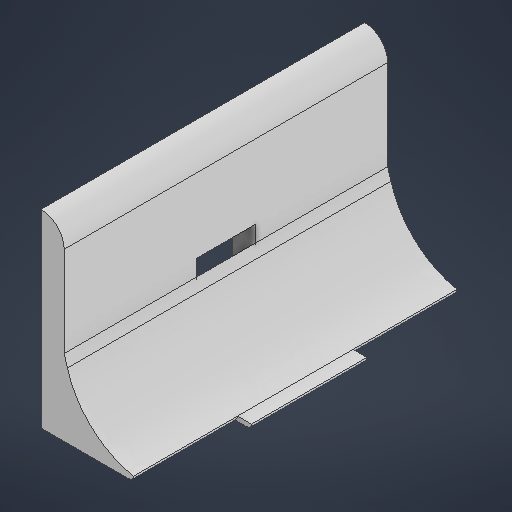
# Autodesk Inventor part: Ramp
Saved by Autodesk Inventor 2026.1 (Build 301233000, 233)
## iProperties
Created: 2026-05-11
Part Number: Ramp
Material: Generic
Document SubType Name: Modeling
Designer: 25adoh
Density: 1 g/cm^3
Appearance: Default
Author: 25adoh
Autodesk Inventor part; units mm, degrees
ref_plane "YZ Plane" through (0, 0, 0) normal (1, 0, 0) x (0, 1, 0)
ref_plane "XZ Plane" through (0, 0, 0) normal (0, 1, 0) x (-1, 0, 0)
ref_plane "XY Plane" through (0, 0, 0) normal (0, 0, 1) x (1, 0, 0)
sketch "Sketch1" plane through (0, 0, 0) normal (1, 0, 0) x (0, 1, 0)
  line L0 (-5, -70) -> (-5, 70)
  line L1 (-5, 70) -> (5, 70)
  line L2 (5, 70) -> (5, -70)
  line L3 (5, -70) -> (-5, -70)
  line L4 (-5, -70) -> (5, 70) construction
  line L5 (-5, 70) -> (5, -70) construction
  line L6 (5, 70) -> (75, 70)
  line L7 (75, 70) -> (75, -70)
  line L8 (75, -70) -> (5, -70)
  line L9 (5, -70) -> (5, 70)
  line L10 (5, -25) -> (5, 0.7)
  line L11 (75, 0.7) -> (75, -25)
  line L12 (35, 12.85) -> (-5, 12.85)
  line L13 (-5, 12.85) -> (-5, -12.85)
  line L14 (-5, -12.85) -> (35, -12.85)
  line L15 (35, -12.85) -> (35, 12.85)
  line L16 (35, 12.85) -> (-5, -12.85) construction
  line L17 (-5, 12.85) -> (35, -12.85) construction
  line L18 (35, -12.85) -> (-10, -12.85)
  line L19 (-10, -12.85) -> (-10, 12.85)
  line L20 (-10, 12.85) -> (35, 12.85)
  line L21 (35, 12.85) -> (35, -12.85)
  point P0 (0, 0)
  point P1 (40, -12.15)
  point P2 (15, 0)
  dimension "d0" = 140
  dimension "d1" = 10
  dimension "d2" = 70
  dimension "d29" = 25.7
  dimension "d30" = 45
  constraints: 44 end point, 9 parallel, 4 midpoint, 4 perpendicular, 3 horizontal, 2 point on line, 1 vertical
  measures "d0" distance of L0.start L0.end
  measures "d1" distance of L0.end L1.end
  measures "d2" distance of L7.end L8.end
  measures "d29" distance of L13.end L12.end
  measures "d30" distance of L19.end L20.end
extrude "Extrusion1" add sketch "Sketch1" along normal blind 10 contours L0 L14 L2 L3 | L0 L12 L2 L14 | L0 L1 L2 L12
extrude "Extrusion2" add sketch "Sketch1" along normal blind 4 contours L2 L14 L15 L12 L6 L7 L8 | L2 L12 L15 L14
extrude "Extrusion3" add sketch "Sketch1" along normal blind 10 contours L2 L14 L15 L12 L6 L7 L8 | L2 L12 L15 L14
sketch "Sketch2" plane through (0, -5, 70) normal (0, 0, 1) x (1, 0, 0)
  line L0 (4, 10) -> (4, 80) projected
  line L1 (10, 0) -> (10, 80) projected
  line L2 (10, 0) -> (20, 0)
  line L3 (10, 10) -> (10, 80) projected
  line L4 (4, 80) -> (4, 0)
  line L5 (4, 0) -> (20, 0)
  line L6 (0, 0) -> (40, 0)
  arc A0 (4, 80) -> (11.3887, 26.2221) centre (170.9276, 75.538) ccw
  arc A1 (11.3887, 26.2221) -> (40, 0) centre (47.0584, 36.4217) ccw
  line L7 (4, 71.0761) -> (4, 0)
  line L8 (4, 0) -> (40, 0)
  line L9 (40, 0) -> (45, 0)
  line L10 (15, 0) -> (25, 0)
  line L11 (9, 0) -> (25, 0)
  line L12 (5, 0) -> (45, 0)
  line L13 (9, 0) -> (45, 0)
  point P0 (0, 5)
  point P1 (10, 38.164)
  point P2 (4, 71.0761)
  point P3 (66.442, 18.3754)
  point P4 (9, 10)
  point P5 (15, 38.164)
  point P6 (15, 10)
  dimension "d11" = 10
  dimension "d15" = 5
  dimension "d16" = 10
  constraints: 22 end point, 5 point on circle, 3 horizontal, 2 centre point, 2 collinear, 2 perpendicular, 2 point on line, 1 vertical
  measures "d11" distance of L1.start L2.end
  measures "d15" distance of L6.end L9.end
  measures "d16" distance of L10.start L10.end
extrude "Extrusion4" add sketch "Sketch2" against normal blind 140 contours L0 A0 L1 L5 L4 | A0 A1 L6 L2 L1
sketch "Sketch3" plane through (4, 75, 25) normal (0, 0, 1) x (1, 0, 0)
  line L0 (6, -70) -> (6, 0)
  line L1 (12, -80) -> (22, -80)
  line L2 (6, 0) -> (6, -80)
  line L3 (6, -80) -> (22, -80)
  line L4 (2, -80) -> (42, -80)
  arc A0 (6, 0) -> (13.3887, -53.7779) centre (172.9276, -4.462) ccw
  arc A1 (13.3887, -53.7779) -> (42, -80) centre (49.0584, -43.5783) ccw
  line L5 (6, -8.9239) -> (6, -80)
  line L6 (6, -80) -> (42, -80)
  line L7 (17, -80) -> (27, -80)
  line L8 (11, -80) -> (27, -80)
  line L9 (7, -80) -> (47, -80)
  line L10 (11, -80) -> (47, -80)
  line L11 (0, 0) -> (0, -8.9239) projected
  line L12 (6, 0) -> (6, -49.0382) projected
  point P0 (-4, -75)
  point P1 (2, -75)
  point P2 (12, -41.836)
  point P3 (68.442, -61.6246)
  point P4 (11, -70)
  point P5 (17, -41.836)
  point P6 (17, -70)
  dimension "d17" = 10
  dimension "d19" = 10
  constraints: 22 end point, 5 point on circle, 2 centre point, 2 collinear, 2 horizontal, 2 perpendicular, 1 point on line, 1 vertical
  measures "d17" distance of L1.start L1.end
  measures "d19" distance of L7.start L7.end
extrude "Extrusion5" [suppressed]
fillet "Fillet1" radius 10 1 edges at (10, 75, 0)
sketch "Sketch4" plane through (0, -5, -70) normal (0, -1, 0) x (1, 0, 0)
  line L0 (0, 140) -> (40, 140) projected
  line L1 (40, 140) -> (0, 140)
  line L2 (0, 140) -> (0, 0)
  line L3 (0, 0) -> (40, 0)
  line L4 (40, 0) -> (40, 140)
  line L5 (17.3887, 95) -> (46, 95) projected
  line L6 (46, 95) -> (40, 95)
  line L7 (40, 95) -> (40, 45)
  line L8 (40, 45) -> (46, 45)
  line L9 (46, 45) -> (46, 95)
  point P0 (0, 70)
  dimension "d23" = 50
  constraints: 16 end point, 4 parallel, 2 horizontal, 2 perpendicular, 1 point on line
  measures "d23" distance of L7.end L6.end
extrude "Extrusion6" add sketch "Sketch4" along normal blind 2
fillet "Fillet2" radius 2 3 edges at (40, -7, 47.5) (46, -7, 0) (40, -7, -47.5)
sketch "Sketch6" plane through (0, 0, 0) normal (-1, 0, 0) x (0, 0, 1)
  line L0 (0, 0) -> (0, -7)
  line L1 (25, -7) -> (-25, -7) projected
  line L2 (12.85, -7) -> (-12.85, -7)
  line L3 (-12.85, -7) -> (12.85, -7)
  line L4 (12.85, -7) -> (12.85, 33)
  line L5 (12.85, 33) -> (-12.85, 33)
  line L6 (-12.85, 33) -> (-12.85, -7)
  dimension "d31" = 25.7
  dimension "d32" = 40
  constraints: 12 end point, 2 midpoint, 2 parallel, 1 horizontal, 1 perpendicular, 1 point on line
  measures "d31" distance of L2.start L2.end
  measures "d32" distance of L4.end L3.end
extrude "Extrusion7" cut sketch "Sketch6" against normal blind 10
body "Solid1"
